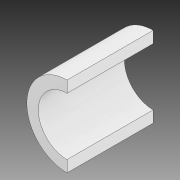
# Autodesk Inventor part: 2101_Tx_Coil_Spacer_v1
Saved by Autodesk Inventor 2021 (Build 250183000, 183)
## iProperties
Created: 2022-06-20
Part Number: 2101_Tx_Coil_Spacer_v1
Material: Acetal Resin, White
Document SubType Name: Modeling
Designer: Eli
Density: 1.425 g/cm^3
Appearance: Smooth - White
Author: Eli
Autodesk Inventor part; units mm, degrees
ref_plane "YZ Plane" through (0, 0, 0) normal (1, 0, 0) x (0, 1, 0)
ref_plane "XZ Plane" through (0, 0, 0) normal (0, 1, 0) x (-1, 0, 0)
ref_plane "XY Plane" through (0, 0, 0) normal (0, 0, 1) x (1, 0, 0)
ref_plane "Work Plane1" through (0, 0, 0) normal (0, 0, 1) x (1, 0, 0)
sketch "Sketch1" plane through (0, 0, 0) normal (0, 0, 1) x (1, 0, 0)
  circle A0 centre (0, 0) radius 14
  circle A1 centre (0, 0) radius 10
  line L0 (0, -14) -> (0, 14)
  point P0 (0, 10)
  point P1 (0, -10)
  dimension "d1" = 4
  dimension "d4" = 20
  constraints: 2 centre point, 2 end point, 2 point on circle, 1 coincident, 1 midpoint, 1 vertical
  measures "d1" radial gap between concentric circles of A0 A1
  measures "d4" diameter of A1
extrude "Extrusion1" add sketch "Sketch1" along normal mid plane 30 contours L0 A1 A0 picked at (-1.9145, -12.4342)
body "Solid1"
